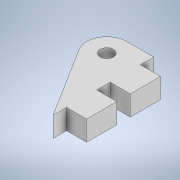
# Autodesk Inventor part: Hinge
Saved by Autodesk Inventor 2020 (Build 240168000, 168)
## iProperties
Created: 2020-07-25
Part Number: Hinge
Material: Generic
Document SubType Name: Modeling
Designer: Aarya
Density: 1 g/cm^3
Appearance: Default
Author: Aarya
Autodesk Inventor part; units mm, degrees
ref_plane "YZ Plane" through (0, 0, 0) normal (1, 0, 0) x (0, 1, 0)
ref_plane "XZ Plane" through (0, 0, 0) normal (0, 1, 0) x (-1, 0, 0)
ref_plane "XY Plane" through (0, 0, 0) normal (0, 0, 1) x (1, 0, 0)
sketch "Sketch1" plane through (0, 0, 0) normal (0, 1, 0) x (-1, 0, 0)
  line L0 (0, 0) -> (3, 0)
  line L1 (3, 0) -> (3, -4.5)
  line L2 (3, -4.5) -> (0, -4.5)
  line L3 (0, -4.5) -> (0, 0)
  line L4 (0, 1) -> (4.5153, 1) construction
  line L5 (0, 2) -> (3, 2)
  line L6 (3, 2) -> (3, 6.5)
  line L7 (3, 6.5) -> (0, 6.5)
  line L8 (0, 6.5) -> (0, 2)
  dimension "d0" = 4.5
  dimension "d1" = 3
  dimension "d2" = 1
  constraints: 18 end point, 4 symmetric about line, 2 parallel, 1 horizontal, 1 perpendicular
  measures "d0" distance of L0.end L1.end
  measures "d1" distance of L1.end L2.end
  measures "d2" distance of L0.start L4.start
extrude "Extrusion1" add sketch "Sketch1" along normal blind 3
sketch "Sketch2" plane through (0, 3, 0) normal (0, 1, 0) x (1, 0, 0)
  line L0 (-3, -8.5) -> (-3, 6.5)
  line L1 (-3, 6.5) -> (-7, 6.5)
  line L2 (-3, -8.5) -> (-9.5398, 1.9034)
  arc A0 (-7, 6.5) -> (-9.5398, 1.9034) centre (-7, 3.5) ccw
  point P0 (0, 0)
  point P1 (-3, -6.5)
  dimension "d5" = 2
  dimension "d6" = 15
  dimension "d10" = 3
  dimension "d11" = 4
  constraints: 6 end point, 2 point on circle, 2 tangent, 1 centre point, 1 horizontal, 1 vertical
  measures "d5" distance of point (-3, -6.5) L0.start
  measures "d6" distance of L0.start L0.end
  measures "d10" radius of A0
  measures "d11" distance of L0.end L1.end
extrude "Extrusion2" add sketch "Sketch2" against normal blind 3
sketch "Sketch3" plane through (0, 3, 0) normal (0, 1, 0) x (1, 0, 0)
  circle A0 centre (-7, 3.5) radius 1
  point P0 (0, 0)
  dimension "d14" = 2
  constraints: 1 centre point, 1 coincident
  measures "d14" diameter of A0
extrude "Extrusion3" cut sketch "Sketch3" against normal blind 3
body "Solid1"
